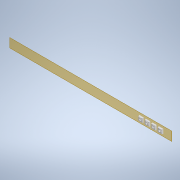
# Autodesk Inventor part: Bottom Holder
Saved by Autodesk Inventor 2022 (Build 260153000, 153)
## iProperties
Created: 2022-03-03
Part Number: Bottom Holder
Material: Generic
Document SubType Name: Modeling
Designer: Nathan Griffith
Density: 1 g/cm^3
Appearance: Default
Author: Nathan Griffith
Autodesk Inventor part; units mm, degrees
ref_plane "YZ Plane" through (0, 0, 0) normal (1, 0, 0) x (0, 1, 0)
ref_plane "XZ Plane" through (0, 0, 0) normal (0, 1, 0) x (-1, 0, 0)
ref_plane "XY Plane" through (0, 0, 0) normal (0, 0, 1) x (1, 0, 0)
ref_plane "Work Plane1" through (0, 0, 0) normal (0, 0, 1) x (1, 0, 0)
ref_plane "Work Plane2" through (0, 0, 0) normal (0, 0, 1) x (1, 0, 0)
ref_plane "Work Plane3" through (0, 0, 0) normal (0, 0, 1) x (1, 0, 0)
sketch "Sketch1" plane through (0, 0, 0) normal (0, 0, 1) x (1, 0, 0)
  line L0 (232.95, -21.7) -> (142.052, -21.7)
  line L1 (142.052, -21.7) -> (142.052, 21.7)
  line L2 (142.052, 21.7) -> (232.95, 21.7)
  line L3 (232.95, 21.7) -> (232.95, -21.7)
  line L4 (148.402, -7.551111) -> (148.402, 7.551111)
  line L5 (226.6, 7.551111) -> (226.6, -7.551111)
  line L6 (205.085111, -9) -> (189.982889, -9)
  line L7 (188.534, 9) -> (206.534, 9)
  circle A0 centre (217.6, 0) radius 2.775
  circle A1 centre (217.6, 0) radius 5.315
  circle A2 centre (197.534, 0) radius 5.315
  circle A3 centre (177.468, 0) radius 5.315
  circle A4 centre (157.402, 0) radius 5.315
  circle A5 centre (217.6, 0) radius 2.775
  circle A6 centre (197.534, 0) radius 2.775
  circle A7 centre (177.468, 0) radius 2.775
  circle A8 centre (157.402, 0) radius 2.775
  line L8 (208.075, 9.906) -> (227.125, 9.906)
  line L9 (227.125, 9.906) -> (227.125, -9.906)
  line L10 (227.125, -9.906) -> (208.075, -9.906)
  line L11 (208.075, -9.906) -> (208.075, 9.906)
  line L12 (208.075, 9.906) -> (227.125, -9.906) construction
  line L13 (227.125, 9.906) -> (208.075, -9.906) construction
  line L14 (207.059, -9.906) -> (188.009, -9.906)
  line L15 (207.059, 9.906) -> (207.059, -9.906)
  line L16 (188.009, 9.906) -> (207.059, 9.906)
  line L17 (188.009, -9.906) -> (188.009, 9.906)
  line L18 (186.993, -9.906) -> (167.943, -9.906)
  line L19 (186.993, 9.906) -> (186.993, -9.906)
  line L20 (167.943, 9.906) -> (186.993, 9.906)
  line L21 (167.943, -9.906) -> (167.943, 9.906)
  line L22 (166.927, -9.906) -> (147.877, -9.906)
  line L23 (166.927, 9.906) -> (166.927, -9.906)
  line L24 (147.877, 9.906) -> (166.927, 9.906)
  line L25 (147.877, -9.906) -> (147.877, 9.906)
  point P0 (0, 0)
  dimension "d0" = 6.35
  dimension "d1" = 6.35
  dimension "d3" = 12.7
  dimension "d4" = 12.7
  dimension "d5" = 2.54
  dimension "d8" = 20.066
  dimension "d15" = 20.066
  dimension "d20" = 19.05
  dimension "d21" = 19.812
  dimension "d24" = 20.066
  constraints: 44 end point, 8 centre point, 5 horizontal, 4 parallel, 2 midpoint, 2 perpendicular, 1 coincident, 1 concentric, 36 other
  measures "d0" distance between parallel lines of L1 L4
  measures "d1" distance between parallel lines of L5 L3
  measures "d3" distance between parallel lines of L0 L6
  measures "d4" distance between parallel lines of L2 L7
  measures "d5" radial gap between concentric circles of A0 A1
  measures "d8" distance of A0.centre A2.centre
  measures "d15" distance of A5.centre A6.centre
  measures "d20" distance of L9.end L10.end
  measures "d21" distance of L8.end L9.end
  measures "d24" distance of L9.end L14.start
extrude "Extrusion1" add sketch "Sketch1" along normal blind 5 contours A1
sketch "Sketch3" plane through (0, 0, 0) normal (0, 0, 1) x (1, 0, 0)
  line L0 (225.6, -8) -> (209.6, -8) projected
  line L1 (225.6, 8) -> (225.6, -8) projected
  line L2 (209.6, 8) -> (225.6, 8) projected
  line L3 (209.6, -8) -> (209.6, 8) projected
  line L4 (210.616, -6.984) -> (224.584, -6.984)
  line L5 (224.584, -6.984) -> (224.584, 6.984)
  line L6 (224.584, 6.984) -> (210.616, 6.984)
  line L7 (210.616, 6.984) -> (210.616, -6.984)
  circle A0 centre (217.6, 0) radius 5.315 projected
  circle A1 centre (217.6, 0) radius 2.775 projected
  point P0 (0, 0)
  dimension "d40" = 1.016
  constraints: 8 end point, 3 other
  measures "d40" distance between parallel lines of L0 L4
sketch "Sketch3 outline for Extrusion3" plane through (0, 0, 0) normal (0, 0, 1) x (1, 0, 0)
  line L0 (210.616, -6.984) -> (224.584, -6.984)
  line L1 (210.616, 6.984) -> (210.616, -6.984)
  line L2 (224.584, -6.984) -> (224.584, 6.984)
  line L3 (224.584, 6.984) -> (210.616, 6.984)
  circle A0 centre (217.6, 0) radius 2.775
extrude "Extrusion3" add sketch "Sketch3 outline for Extrusion3" along normal blind 4 draft -15
pattern_linear "Rectangular Pattern1" count 4 spacing 20.066 along (-1, 0, 0) of "Extrusion3", "Extrusion1"
ref_plane "Work Plane4" through (0, 0, 0) normal (0, 0, 1) x (1, 0, 0)
sketch "Sketch4" plane through (0, 0, 0) normal (0, 0, 1) x (1, 0, 0)
  line L0 (-228.6, 12.7) -> (228.6, 12.7) projected
  line L1 (228.6, -12.7) -> (-228.6, -12.7) projected
  line L2 (228.6, 12.7) -> (228.6, -12.7) projected
  line L3 (146.336, 9) -> (146.336, -9) projected
  line L4 (228.6, 12.7) -> (146.336, 12.7)
  line L5 (146.336, 12.7) -> (146.336, -12.7)
  line L6 (146.336, -12.7) -> (228.6, -12.7)
  line L7 (228.6, -12.7) -> (228.6, 12.7)
  point P0 (0, 0)
  constraints: 8 end point, 2 parallel, 2 point on line, 1 horizontal, 1 perpendicular
extrude "Extrusion4" add sketch "Sketch4" against normal blind 4
body "Solid1"
